Autodesk Inventor part; units mm, degrees
(part 6 of 6)
  line L4434 (21.6889, 20.6189) -> (21.8877, 20.7047)
  line L4435 (21.8877, 20.7047) -> (22.099, 20.7906)
  line L4436 (22.099, 20.7906) -> (22.3249, 20.8771)
  line L4437 (22.3249, 20.8771) -> (22.5632, 20.9626)
  line L4438 (22.5632, 20.9626) -> (22.7728, 21.0333)
  arc A141 (23.2985, 20.4495) -> (22.7728, 21.0333) centre (0, 0) ccw
  line L4439 (23.2985, 20.4495) -> (23.2063, 20.2484)
  line L4440 (23.2063, 20.2484) -> (23.0963, 20.0203)
  line L4441 (23.0963, 20.0203) -> (22.9867, 19.8047)
  line L4442 (22.9867, 19.8047) -> (22.8791, 19.6036)
  line L4443 (22.8791, 19.6036) -> (22.773, 19.4148)
  line L4444 (22.773, 19.4148) -> (22.6688, 19.2381)
  line L4445 (22.6688, 19.2381) -> (22.5683, 19.0757)
  line L4446 (22.5683, 19.0757) -> (22.4708, 18.9253)
  line L4447 (22.4708, 18.9253) -> (22.2724, 18.6353)
  line L4448 (22.2724, 18.6353) -> (22.2519, 18.5933)
  line L4449 (22.2519, 18.5933) -> (22.2427, 18.5587)
  line L4450 (22.2427, 18.5587) -> (22.2446, 18.5322)
  line L4451 (22.2446, 18.5322) -> (22.2531, 18.5178)
  line L4452 (22.2531, 18.5178) -> (22.4984, 18.2188)
  line L4453 (22.4984, 18.2188) -> (22.7398, 17.9167)
  line L4454 (22.7398, 17.9167) -> (22.7521, 17.9055)
  line L4455 (22.7521, 17.9055) -> (22.7777, 17.8981)
  line L4456 (22.7777, 17.8981) -> (22.8134, 17.8999)
  line L4457 (22.8134, 17.8999) -> (22.8588, 17.9112)
  line L4458 (22.8588, 17.9112) -> (23.1837, 18.045)
  line L4459 (23.1837, 18.045) -> (23.3511, 18.1091)
  line L4460 (23.3511, 18.1091) -> (23.5308, 18.1736)
  line L4461 (23.5308, 18.1736) -> (23.7253, 18.2388)
  line L4462 (23.7253, 18.2388) -> (23.932, 18.3034)
  line L4463 (23.932, 18.3034) -> (24.1511, 18.3668)
  line L4464 (24.1511, 18.3668) -> (24.3848, 18.4292)
  line L4465 (24.3848, 18.4292) -> (24.6308, 18.4893)
  line L4466 (24.6308, 18.4893) -> (24.8466, 18.5377)
  arc A142 (25.3084, 17.9021) -> (24.8466, 18.5377) centre (0, 0) ccw
  line L4467 (25.3084, 17.9021) -> (25.1957, 17.7118)
  line L4468 (25.1957, 17.7118) -> (25.0625, 17.4964)
  line L4469 (25.0625, 17.4964) -> (24.931, 17.2934)
  line L4470 (24.931, 17.2934) -> (24.8029, 17.1047)
  line L4471 (24.8029, 17.1047) -> (24.6777, 16.928)
  line L4472 (24.6777, 16.928) -> (24.5555, 16.7632)
  line L4473 (24.5555, 16.7632) -> (24.4386, 16.6122)
  line L4474 (24.4386, 16.6122) -> (24.326, 16.4728)
  line L4475 (24.326, 16.4728) -> (24.0984, 16.2052)
  line L4476 (24.0984, 16.2052) -> (24.0735, 16.1655)
  line L4477 (24.0735, 16.1655) -> (24.0608, 16.1321)
  line L4478 (24.0608, 16.1321) -> (24.0599, 16.1055)
  line L4479 (24.0599, 16.1055) -> (24.0668, 16.0903)
  line L4480 (24.0668, 16.0903) -> (24.2795, 15.7673)
  line L4481 (24.2795, 15.7673) -> (24.488, 15.4416)
  line L4482 (24.488, 15.4416) -> (24.4991, 15.4291)
  line L4483 (24.4991, 15.4291) -> (24.5238, 15.4191)
  line L4484 (24.5238, 15.4191) -> (24.5595, 15.4172)
  line L4485 (24.5595, 15.4172) -> (24.6058, 15.4237)
  line L4486 (24.6058, 15.4237) -> (24.9429, 15.5228)
  line L4487 (24.9429, 15.5228) -> (25.1161, 15.569)
  line L4488 (25.1161, 15.569) -> (25.3015, 15.6144)
  line L4489 (25.3015, 15.6144) -> (25.5018, 15.6589)
  line L4490 (25.5018, 15.6589) -> (25.7142, 15.7015)
  line L4491 (25.7142, 15.7015) -> (25.9387, 15.7417)
  line L4492 (25.9387, 15.7417) -> (26.1776, 15.7793)
  line L4493 (26.1776, 15.7793) -> (26.4285, 15.8134)
  line L4494 (26.4285, 15.8134) -> (26.6482, 15.8389)
  arc A143 (27.041, 15.1586) -> (26.6482, 15.8389) centre (0, 0) ccw
  line L4495 (27.041, 15.1586) -> (26.9091, 14.9811)
  line L4496 (26.9091, 14.9811) -> (26.7541, 14.7808)
  line L4497 (26.7541, 14.7808) -> (26.602, 14.5927)
  line L4498 (26.602, 14.5927) -> (26.455, 14.4184)
  line L4499 (26.455, 14.4184) -> (26.312, 14.2558)
  line L4500 (26.312, 14.2558) -> (26.1732, 14.1046)
  line L4501 (26.1732, 14.1046) -> (26.0412, 13.9666)
  line L4502 (26.0412, 13.9666) -> (25.9146, 13.8398)
  line L4503 (25.9146, 13.8398) -> (25.6603, 13.5974)
  line L4504 (25.6603, 13.5974) -> (25.6314, 13.5605)
  line L4505 (25.6314, 13.5605) -> (25.6153, 13.5287)
  line L4506 (25.6153, 13.5287) -> (25.6116, 13.5023)
  line L4507 (25.6116, 13.5023) -> (25.6168, 13.4865)
  line L4508 (25.6168, 13.4865) -> (25.7946, 13.143)
  line L4509 (25.7946, 13.143) -> (25.968, 12.7973)
  line L4510 (25.968, 12.7973) -> (25.9777, 12.7837)
  line L4511 (25.9777, 12.7837) -> (26.0012, 12.7712)
  line L4512 (26.0012, 12.7712) -> (26.0365, 12.7656)
  line L4513 (26.0365, 12.7656) -> (26.0833, 12.7672)
  line L4514 (26.0833, 12.7672) -> (26.4288, 12.8305)
  line L4515 (26.4288, 12.8305) -> (26.6059, 12.8584)
  line L4516 (26.6059, 12.8584) -> (26.7951, 12.8841)
  line L4517 (26.7951, 12.8841) -> (26.9989, 12.9075)
  line L4518 (26.9989, 12.9075) -> (27.2145, 12.9276)
  line L4519 (27.2145, 12.9276) -> (27.442, 12.9441)
  line L4520 (27.442, 12.9441) -> (27.6836, 12.9565)
  line L4521 (27.6836, 12.9565) -> (27.9367, 12.9642)
  line L4522 (27.9367, 12.9642) -> (28.1579, 12.9667)
  arc A144 (28.4774, 12.249) -> (28.1579, 12.9667) centre (0, 0) ccw
  line L4523 (28.4774, 12.249) -> (28.3276, 12.0862)
  line L4524 (28.3276, 12.0862) -> (28.1525, 11.9033)
  line L4525 (28.1525, 11.9033) -> (27.9817, 11.7321)
  line L4526 (27.9817, 11.7321) -> (27.8172, 11.5741)
  line L4527 (27.8172, 11.5741) -> (27.6579, 11.4273)
  line L4528 (27.6579, 11.4273) -> (27.5042, 11.2915)
  line L4529 (27.5042, 11.2915) -> (27.3584, 11.1681)
  line L4530 (27.3584, 11.1681) -> (27.2193, 11.0551)
  line L4531 (27.2193, 11.0551) -> (26.941, 10.8407)
  line L4532 (26.941, 10.8407) -> (26.9085, 10.807)
  line L4533 (26.9085, 10.807) -> (26.8891, 10.777)
  line L4534 (26.8891, 10.777) -> (26.8826, 10.7512)
  line L4535 (26.8826, 10.7512) -> (26.8862, 10.7349)
  line L4536 (26.8862, 10.7349) -> (27.0272, 10.3748)
  line L4537 (27.0272, 10.3748) -> (27.1634, 10.0128)
  line L4538 (27.1634, 10.0128) -> (27.1717, 9.9983)
  line L4539 (27.1717, 9.9983) -> (27.1937, 9.9834)
  line L4540 (27.1937, 9.9834) -> (27.2282, 9.9741)
  line L4541 (27.2282, 9.9741) -> (27.2749, 9.9708)
  line L4542 (27.2749, 9.9708) -> (27.6252, 9.9977)
  line L4543 (27.6252, 9.9977) -> (27.8042, 10.0069)
  line L4544 (27.8042, 10.0069) -> (27.995, 10.0127)
  line L4545 (27.995, 10.0127) -> (28.2002, 10.0146)
  line L4546 (28.2002, 10.0146) -> (28.4168, 10.0121)
  line L4547 (28.4168, 10.0121) -> (28.6447, 10.0047)
  line L4548 (28.6447, 10.0047) -> (28.8863, 9.9918)
  line L4549 (28.8863, 9.9918) -> (29.1388, 9.973)
  line L4550 (29.1388, 9.973) -> (29.359, 9.9523)
  arc A145 (29.6018, 9.2052) -> (29.359, 9.9523) centre (0, 0) ccw
  line L4551 (29.6018, 9.2052) -> (29.4358, 9.059)
  line L4552 (29.4358, 9.059) -> (29.2425, 8.8954)
  line L4553 (29.2425, 8.8954) -> (29.0547, 8.7429)
  line L4554 (29.0547, 8.7429) -> (28.8746, 8.603)
  line L4555 (28.8746, 8.603) -> (28.7009, 8.4737)
  line L4556 (28.7009, 8.4737) -> (28.5338, 8.3547)
  line L4557 (28.5338, 8.3547) -> (28.3759, 8.2472)
  line L4558 (28.3759, 8.2472) -> (28.2257, 8.1494)
  line L4559 (28.2257, 8.1494) -> (27.9266, 7.9652)
  line L4560 (27.9266, 7.9652) -> (27.8907, 7.9351)
  line L4561 (27.8907, 7.9351) -> (27.8683, 7.9073)
  line L4562 (27.8683, 7.9073) -> (27.8592, 7.8823)
  line L4563 (27.8592, 7.8823) -> (27.861, 7.8657)
  line L4564 (27.861, 7.8657) -> (27.9636, 7.4928)
  line L4565 (27.9636, 7.4928) -> (28.0612, 7.1186)
  line L4566 (28.0612, 7.1186) -> (28.0679, 7.1033)
  line L4567 (28.0679, 7.1033) -> (28.0883, 7.0862)
  line L4568 (28.0883, 7.0862) -> (28.1216, 7.0733)
  line L4569 (28.1216, 7.0733) -> (28.1677, 7.0652)
  line L4570 (28.1677, 7.0652) -> (28.5189, 7.0553)
  line L4571 (28.5189, 7.0553) -> (28.6979, 7.0457)
  line L4572 (28.6979, 7.0457) -> (28.8883, 7.0315)
  line L4573 (28.8883, 7.0315) -> (29.0926, 7.012)
  line L4574 (29.0926, 7.012) -> (29.3077, 6.9869)
  line L4575 (29.3077, 6.9869) -> (29.5336, 6.9557)
  line L4576 (29.5336, 6.9557) -> (29.7725, 6.9177)
  line L4577 (29.7725, 6.9177) -> (30.0216, 6.8726)
  line L4578 (30.0216, 6.8726) -> (30.2385, 6.829)
  arc A146 (30.4018, 6.0605) -> (30.2385, 6.829) centre (0, 0) ccw
  line L4579 (30.4018, 6.0605) -> (30.2214, 5.9325)
  line L4580 (30.2214, 5.9325) -> (30.0122, 5.79)
  line L4581 (30.0122, 5.79) -> (29.8094, 5.658)
  line L4582 (29.8094, 5.658) -> (29.6157, 5.5376)
  line L4583 (29.6157, 5.5376) -> (29.4294, 5.4272)
  line L4584 (29.4294, 5.4272) -> (29.2508, 5.3263)
  line L4585 (29.2508, 5.3263) -> (29.0826, 5.2359)
  line L4586 (29.0826, 5.2359) -> (28.9229, 5.1544)
  line L4587 (28.9229, 5.1544) -> (28.6062, 5.0025)
  line L4588 (28.6062, 5.0025) -> (28.5674, 4.9763)
  line L4589 (28.5674, 4.9763) -> (28.5421, 4.951)
  line L4590 (28.5421, 4.951) -> (28.5305, 4.927)
  line L4591 (28.5305, 4.927) -> (28.5306, 4.9104)
  line L4592 (28.5306, 4.9104) -> (28.5936, 4.5288)
  line L4593 (28.5936, 4.5288) -> (28.6516, 4.1464)
  line L4594 (28.6516, 4.1464) -> (28.6567, 4.1305)
  line L4595 (28.6567, 4.1305) -> (28.6751, 4.1114)
  line L4596 (28.6751, 4.1114) -> (28.7069, 4.0951)
  line L4597 (28.7069, 4.0951) -> (28.7519, 4.0822)
  line L4598 (28.7519, 4.0822) -> (29.1001, 4.0356)
  line L4599 (29.1001, 4.0356) -> (29.2771, 4.0074)
  line L4600 (29.2771, 4.0074) -> (29.465, 3.9734)
  line L4601 (29.465, 3.9734) -> (29.6661, 3.9326)
  line L4602 (29.6661, 3.9326) -> (29.8774, 3.8852)
  line L4603 (29.8774, 3.8852) -> (30.0989, 3.8305)
  line L4604 (30.0989, 3.8305) -> (30.3325, 3.7677)
  line L4605 (30.3325, 3.7677) -> (30.5755, 3.6968)
  line L4606 (30.5755, 3.6968) -> (30.7866, 3.6308)
  arc A147 (30.8688, 2.8495) -> (30.7866, 3.6308) centre (0, 0) ccw
  line L4607 (30.8688, 2.8495) -> (30.676, 2.741)
  point P0 (30.8358, -4.7255)
  point P1 (31.2745, -5.1642)
  point P2 (33.8904, -6.6745)
  point P3 (34.4897, -6.8351)
  point P4 (37.5103, -6.8351)
  point P5 (38.1096, -6.6745)
  point P6 (40.7255, -5.1642)
  point P7 (41.1642, -4.7255)
  point P8 (42.6745, -2.1096)
  point P9 (42.8351, -1.5103)
  point P10 (42.8351, 1.5103)
  point P11 (42.6745, 2.1096)
  point P12 (41.1642, 4.7255)
  point P13 (40.7255, 5.1642)
  point P14 (38.1096, 6.6745)
  point P15 (37.5103, 6.8351)
  point P16 (34.4897, 6.8351)
  point P17 (33.8904, 6.6745)
  point P18 (31.2745, 5.1642)
  point P19 (30.8358, 4.7255)
  point P20 (29.3255, 2.1096)
  point P21 (29.1649, 1.5103)
  point P22 (29.1649, -1.5103)
  point P23 (29.3255, -2.1096)
  point P24 (30.8688, 2.8495)
  point P25 (30.7866, 3.6308)
  point P26 (30.4018, 6.0605)
  point P27 (30.2385, 6.829)
  point P28 (29.6018, 9.2052)
  point P29 (29.359, 9.9523)
  point P30 (28.4774, 12.249)
  point P31 (28.1579, 12.9667)
  point P32 (27.041, 15.1586)
  point P33 (26.6482, 15.8389)
  point P34 (25.3084, 17.9021)
  point P35 (24.8466, 18.5377)
  point P36 (23.2985, 20.4495)
  point P37 (22.7728, 21.0333)
  point P38 (21.0333, 22.7728)
  point P39 (20.4495, 23.2985)
  point P40 (18.5377, 24.8466)
  point P41 (17.9021, 25.3084)
  point P42 (15.8389, 26.6482)
  point P43 (15.1586, 27.041)
  point P44 (12.9667, 28.1579)
  point P45 (12.249, 28.4774)
  point P46 (9.9523, 29.359)
  point P47 (9.2052, 29.6018)
  point P48 (6.0605, 30.4018)
  point P49 (3.6308, 30.7866)
  point P50 (2.8495, 30.8688)
  point P51 (0.3928, 30.9975)
  point P52 (-0.3928, 30.9975)
  point P53 (-2.8495, 30.8688)
  point P54 (-3.6308, 30.7866)
  point P55 (-6.0605, 30.4018)
  point P56 (-6.829, 30.2385)
  point P57 (-9.2052, 29.6018)
  point P58 (-9.9523, 29.359)
  point P59 (-12.249, 28.4774)
  point P60 (-12.9667, 28.1579)
  point P61 (-15.1586, 27.041)
  point P62 (-15.8389, 26.6482)
  point P63 (-17.9021, 25.3084)
  point P64 (-18.5377, 24.8466)
  point P65 (-20.4495, 23.2985)
  point P66 (-21.0333, 22.7728)
  point P67 (-22.7728, 21.0333)
  point P68 (-23.2985, 20.4495)
  point P69 (-24.8466, 18.5377)
  point P70 (-25.3084, 17.9021)
  point P71 (-26.6482, 15.8389)
  point P72 (-27.041, 15.1586)
  point P73 (-28.1579, 12.9667)
  point P74 (-28.4774, 12.249)
  point P75 (-29.359, 9.9523)
  point P76 (-29.6018, 9.2052)
  point P77 (-30.4018, 6.0605)
  point P78 (-30.7866, 3.6308)
  point P79 (-30.8688, 2.8495)
  point P80 (-30.9975, 0.3928)
  point P81 (-30.9975, -0.3928)
  point P82 (-30.8688, -2.8495)
  point P83 (-30.7866, -3.6308)
  point P84 (-30.4018, -6.0605)
  point P85 (-30.2385, -6.829)
  point P86 (-29.6018, -9.2052)
  point P87 (-29.359, -9.9523)
  point P88 (-28.4774, -12.249)
  point P89 (-28.1579, -12.9667)
  point P90 (-27.041, -15.1586)
  point P91 (-26.6482, -15.8389)
  point P92 (-25.3084, -17.9021)
  point P93 (-24.8466, -18.5377)
  point P94 (-23.2985, -20.4495)
  point P95 (-22.7728, -21.0333)
  point P96 (-21.0333, -22.7728)
  point P97 (-20.4495, -23.2985)
  point P98 (-18.5377, -24.8466)
  point P99 (-17.9021, -25.3084)
  point P100 (-15.8389, -26.6482)
  point P101 (-15.1586, -27.041)
  point P102 (-12.9667, -28.1579)
  point P103 (-12.249, -28.4774)
  point P104 (-9.9523, -29.359)
  point P105 (-9.2052, -29.6018)
  point P106 (-6.829, -30.2385)
  point P107 (-6.0605, -30.4018)
  point P108 (-3.6308, -30.7866)
  point P109 (-2.8495, -30.8688)
  point P110 (-0.3928, -30.9975)
  point P111 (0.3928, -30.9975)
  point P112 (2.8495, -30.8688)
  point P113 (3.6308, -30.7866)
  point P114 (6.0605, -30.4018)
  point P115 (6.829, -30.2385)
  point P116 (9.2052, -29.6018)
  point P117 (9.9523, -29.359)
  point P118 (12.249, -28.4774)
  point P119 (12.9667, -28.1579)
  point P120 (15.1586, -27.041)
  point P121 (15.8389, -26.6482)
  point P122 (17.9021, -25.3084)
  point P123 (18.5377, -24.8466)
  point P124 (20.4495, -23.2985)
  point P125 (21.0333, -22.7728)
  point P126 (22.7728, -21.0333)
  point P127 (23.2985, -20.4495)
  point P128 (24.8466, -18.5377)
  point P129 (25.3084, -17.9021)
  point P130 (26.6482, -15.8389)
  point P131 (27.041, -15.1586)
  point P132 (28.1579, -12.9667)
  point P133 (28.4774, -12.249)
  point P134 (29.359, -9.9523)
  point P135 (29.6018, -9.2052)
  point P136 (30.2385, -6.829)
  point P137 (30.4018, -6.0605)
  point P138 (30.7866, -3.6308)
  point P139 (30.8688, -2.8495)
  point P140 (30.9975, -0.3928)
  point P141 (30.9975, 0.3928)
  constraints: 9216 end point, 288 point on circle, 148 centre point
extrude "Extrusion1" add sketch "Sketch1" along normal blind 6.2 contours L0 L1 L2 L3 L4 L5 L6 L7 L8 L9 L10 L11 L12 L13 L14 L15 L16 L17 L18 L19 L20 L21 L22 L23 L24 L25 L26 L27 L28 L29 L30 L31 L32 L33 L34 L35 L36 L37 L38 L39 L40 L41 L42 L43 L44 L45 L46 L47 L48 L49 L50 A4 L51 L52 L53 L54 L55 L56 L57 L58 L59 L60 L61 L62 L63 L64 L65 L66 L67 L68 L69 L70 L71 L72 L73 L74 L75 L76 L77 L78 L79 L80 L81 L82 L83 L84 L85 L86 L87 L88 L89 L90 L91 L92 L93 L94 L95 L96 L97 L98 L99 L100 L101 L102 A5 L103 L104 L105 L106 L107 L108 L109 L110 L111 L112 L113 L114 L115 L116 L117 L118 L119 L120 L121 L122 L123 L124 L125 L126 L127 L128 L129 L130 L131 L132 L133 L134 L135 L136 L137 L138 L139 L140 L141 L142 L143 L144 L145 L146 L147 L148 L149 L150 L151 L152 L153 L154 A6 L155 L156 L157 L158 L159 L160 L161 L162 L163 L164 L165 L166 L167 L168 L169 L170 L171 L172 L173 L174 L175 L176 L177 L178 L179 L180 L181 L182 L183 L184 L185 L186 L187 L188 L189 L190 L191 L192 L193 L194 L195 L196 L197 L198 L199 L200 L201 L202 L203 L204 L205 L206 A7 L207 L208 L209 L210 L211 L212 L213 L214 L215 L216 L217 L218 L219 L220 L221 L222 L223 L224 L225 L226 L227 L228 L229 L230 L231 L232 L233 L234 L235 L236 L237 L238 L239 L240 L241 L242 L243 L244 L245 L246 L247 L248 L249 L250 L251 L252 L253 L254 L255 L256 L257 L258 A8 L259 L260 L261 L262 L263 L264 L265 L266 L267 L268 L269 L270 L271 L272 L273 L274 L275 L276 L277 L278 L279 L280 L281 L282 L283 L284 L285 L286 L287 L288 L289 L290 L291 L292 L293 L294 L295 L296 L297 L298 L299 L300 L301 L302 L303 L304 L305 L306 L307 L308 L309 L310 A9 L311 L312 L313 L314 L315 L316 L317 L318 L319 L320 L321 L322 L323 L324 L325 L326 L327 L328 L329 L330 L331 L332 L333 L334 L335 L336 L337 L338 L339 L340 L341 L342 L343 L344 L345 L346 L347 L348 L349 L350 L351 L352 L353 L354 L355 L356 L357 L358 L359 L360 L361 L362 A10 L363 L364 L365 L366 L367 L368 L369 L370 L371 L372 L373 L374 L375 L376 L377 L378 L379 L380 L381 L382 L383 L384 L385 L386 L387 L388 L389 L390 L391 L392 L393 L394 L395 L396 L397 L398 L399 L400 L401 L402 L403 L404 L405 L406 L407 L408 L409 L410 L411 L412 L413 L414 A11 L415 L416 L417 L418 L419 L420 L421 L422 L423 L424 L425 L426 L427 L428 L429 L430 L431 L432 L433 L434 L435 L436 L437 L438 L439 L440 L441 L442 L443 L444 L445 L446 L447 L448 L449 L450 L451 L452 L453 L454 L455 L456 L457 L458 L459 L460 L461 L462 L463 L464 L465 L466 A12 L467 L468 L469 L470 L471 L472 L473 L474 L475 L476 L477 L478 L479 L480 L481 L482 L483 L484 L485 L486 L487 L488 L489 L490 L491 L492 L493 L494 L495 L496 L497 L498 L499 L500 L501 L502 L503 L504 L505 L506 L507 L508 L509 L510 L511 L512 L513 L514 L515 L516 L517 L518 A13 L519 L520 L521 L522 L523 L524 L525 L526 L527 L528 L529 L530 L531 L532 L533 L534 L535 L536 L537 L538 L539 L540 L541 L542 L543 L544 L545 L546 L547 L548 L549 L550 L551 L552 L553 L554 L555 L556 L557 L558 L559 L560 L561 L562 L563 L564 L565 L566 L567 L568 L569 L570 A14 L571 L572 L573 L574 L575 L576 L577 L578 L579 L580 L581 L582 L583 L584 L585 L586 L587 L588 L589 L590 L591 L592 L593 L594 L595 L596 L597 L598 L599 L600 L601 L602 L603 L604 L605 L606 L607 L608 L609 L610 L611 L612 L613 L614 L615 L616 L617 L618 L619 L620 L621 L622 A15 L623
sketch "Sketch4" plane through (0, 0, 6.2) normal (0, 0, 1) x (1, 0, 0)
  circle A0 centre (36, 0) radius 2 projected
  line L0 (36, 0) -> (39.1, 0) construction
  line L1 (36, 0) -> (37.55, 2.6847) construction
  line L2 (36, 0) -> (34.45, 2.6847) construction
  line L3 (36, 0) -> (32.9, 0) construction
  line L4 (36, 0) -> (34.45, -2.6847) construction
  line L5 (36, 0) -> (37.55, -2.6847) construction
  line L6 (34.45, 2.6847) -> (37.55, 2.6847) construction
  line L7 (37.55, 2.6847) -> (39.1, 0) construction
  line L8 (39.1, 0) -> (37.55, -2.6847) construction
  line L9 (37.55, -2.6847) -> (34.45, -2.6847) construction
  line L10 (34.45, -2.6847) -> (32.9, 0) construction
  line L11 (32.9, 0) -> (34.45, 2.6847) construction
  line L12 (39.6774, 0) -> (37.8387, 3.1847)
  line L13 (37.8387, 3.1847) -> (34.1613, 3.1847)
  line L14 (34.1613, 3.1847) -> (32.3226, 0)
  line L15 (32.3226, 0) -> (34.1613, -3.1847)
  line L16 (34.1613, -3.1847) -> (37.8387, -3.1847)
  line L17 (37.8387, -3.1847) -> (39.6774, 0)
  point P0 (0, 0)
  dimension "d30" = 3.1
  dimension "d33" = 360
  dimension "d37" = 0.5
  constraints: 36 end point, 6 parallel, 2 coincident, 2 horizontal, 22 other
  measures "d30" distance of L0.start L0.end
  measures "d37" distance between parallel lines of L7 L12
extrude "Extrusion8" cut sketch "Sketch4" against normal blind 10
body "Solid1"
